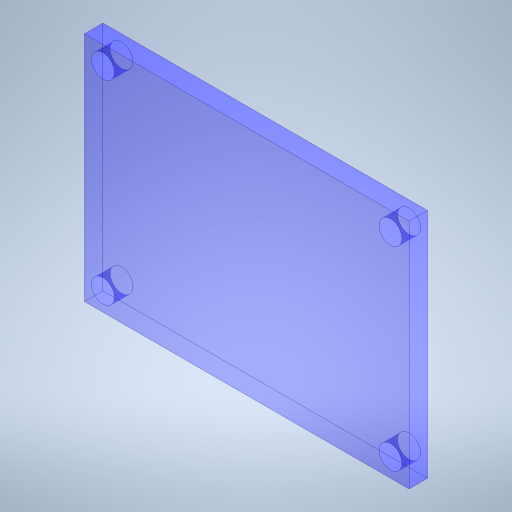
# Autodesk Inventor part: acrylic
Saved by Autodesk Inventor 2024.2 (Build 282272000, 272)
## iProperties
Created: 2022-02-08
Part Number: acrylic
Material: Generic
Document SubType Name: Modeling
Designer: magoo
Density: 1 g/cm^3
Appearance: Default
Description: Acrylic sheet cut
Author: magoo
Autodesk Inventor part; units mm, degrees
ref_plane "YZ Plane" through (0, 0, 0) normal (1, 0, 0) x (0, 1, 0)
ref_plane "XZ Plane" through (0, 0, 0) normal (0, 1, 0) x (-1, 0, 0)
ref_plane "XY Plane" through (0, 0, 0) normal (0, 0, 1) x (1, 0, 0)
sketch "Sketch1" plane through (0, 0, 0) normal (0, 0, 1) x (1, 0, 0)
  line L0 (17.5, -12.5) -> (-17.5, -12.5)
  line L1 (-17.5, -12.5) -> (-17.5, 12.5)
  line L2 (-17.5, 12.5) -> (17.5, 12.5)
  line L3 (17.5, 12.5) -> (17.5, -12.5)
  line L4 (17.5, -12.5) -> (-17.5, 12.5) construction
  line L5 (-17.5, -12.5) -> (17.5, 12.5) construction
  circle A0 centre (-15.5, 10.5) radius 1.25
  circle A1 centre (15.5, 10.5) radius 1.25
  circle A2 centre (-15.5, -10.5) radius 1.25
  circle A3 centre (15.5, -10.5) radius 1.25
  point P0 (0, 0)
  dimension "d0" = 25
  dimension "d1" = 35
  dimension "d2" = 2
  dimension "d3" = 2
  dimension "d4" = 2
  dimension "d5" = 2
  dimension "d6" = 2
  dimension "d7" = 2
  dimension "d8" = 2
  dimension "d9" = 2
  dimension "d10" = 2.5
  dimension "d11" = 2.5
  dimension "d12" = 2.5
  dimension "d13" = 2.5
  constraints: 12 end point, 4 centre point, 2 midpoint, 2 parallel, 1 horizontal, 1 perpendicular
  measures "d0" distance of L0.end L1.end
  measures "d1" distance of L1.end L2.end
  measures "d2" distance from line of L2 A0.centre
  measures "d3" distance from line of L1 A0.centre
  measures "d4" distance from line of L3 A1.centre
  measures "d5" distance from line of L2 A1.centre
  measures "d6" distance from line of L1 A2.centre
  measures "d7" distance from line of L0 A2.centre
  measures "d8" distance from line of L3 A3.centre
  measures "d9" distance from line of L0 A3.centre
  measures "d10" diameter of A1
  measures "d11" diameter of A3
  measures "d12" diameter of A0
  measures "d13" diameter of A2
extrude "Extrusion1" add sketch "Sketch1" along normal blind 2
body "Solid1"
